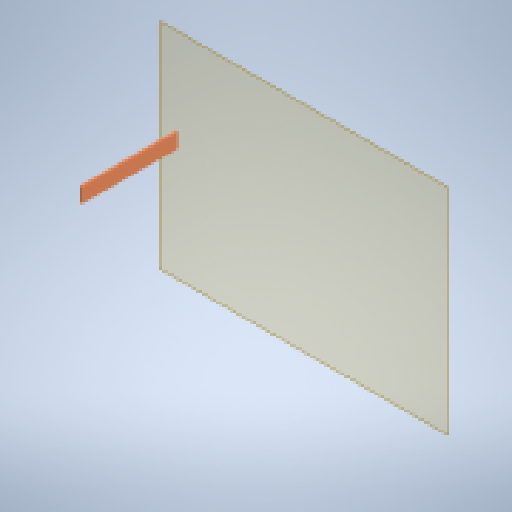
# Autodesk Inventor part: PuertaPequeña
Saved by Autodesk Inventor 2024 (Build 280153000, 153)
## iProperties
Created: 2024-04-05
Part Number: PuertaPequeña
Material: Genérico
Document SubType Name: Modeling
Designer: sergi
Density: 1 g/cm^3
Appearance: Valor por defecto
Author: sergi
Autodesk Inventor part; units mm, degrees
ref_plane "YZ Plane" through (0, 0, 0) normal (1, 0, 0) x (0, 1, 0)
ref_plane "XZ Plane" through (0, 0, 0) normal (0, 1, 0) x (-1, 0, 0)
ref_plane "Plano de trabajo1" through (0, 0, 0) normal (0, 0, 1) x (1, 0, 0)
sketch "Boceto1" plane through (0, 0, 0) normal (0, 0, 1) x (1, 0, 0)
  line L0 (-2650.7331, 1162.5) -> (-2750.7331, 1162.5) projected
  line L1 (-2650.7331, 132.5) -> (-2650.7331, 1162.5) projected
  line L2 (-2750.7331, 132.5) -> (-2650.7331, 132.5) projected
  line L3 (-2750.7331, 132.5) -> (-2750.7331, 1162.5) projected
  line L4 (-2650.7331, 132.5) -> (-2700.7331, 132.5)
  line L5 (-2700.7331, 132.5) -> (-2700.7331, 442.5)
  line L6 (-2700.7331, 442.5) -> (-2650.7331, 442.5)
  line L7 (-2650.7331, 442.5) -> (-2650.7331, 132.5)
  point P0 (0, 0)
  dimension "d0" = 310
  constraints: 8 end point, 2 parallel, 1 horizontal, 1 perpendicular
  measures "d0" distance of L4.end L5.end
ref_plane "Plano de trabajo2" through (-2750.7331, 132.5, 2030) normal (0, 0, -1) x (0, 1, 0)
extrude "Extrusión1" add sketch "Boceto1" along normal up to surface (2030 mm away) contours L1 L2 L5 L6
